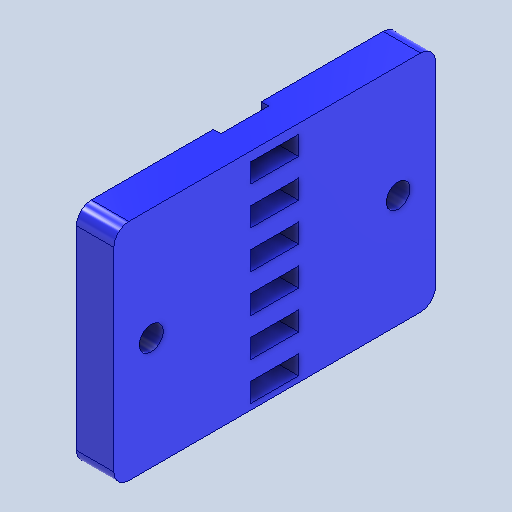
# Autodesk Inventor part: dribl-v3-3DP-3
Saved by Autodesk Inventor 2025.2 (Build 292293000, 293)
## iProperties
Created: 2025-04-20
Part Number: dribl-v3-3DP-3
Material: ABS プラスチック
Document SubType Name: Modeling
Designer: haruy
Density: 1.06 g/cm^3
Appearance: 青 - 壁塗料 - 光沢
Author: haruy
Autodesk Inventor part; units mm, degrees
ref_plane "YZ Plane" through (0, 0, 0) normal (1, 0, 0) x (0, 1, 0)
ref_plane "XZ Plane" through (0, 0, 0) normal (0, 1, 0) x (-1, 0, 0)
ref_plane "XY Plane" through (0, 0, 0) normal (0, 0, 1) x (1, 0, 0)
sketch "スケッチ1" plane through (0, 0, 0) normal (1, 0, 0) x (0, 1, 0)
  line L0 (0, 0) -> (30, 0)
  line L1 (30, 0) -> (30, -43)
  line L2 (30, -43) -> (0, -43)
  line L3 (0, -43) -> (0, 0)
  circle A0 centre (15, -5) radius 1.6
  circle A1 centre (15, -38) radius 1.6
  line L4 (28.75, -18.3) -> (26.18, -18.3)
  line L5 (26.18, -18.3) -> (26.18, -24.7)
  line L6 (26.18, -24.7) -> (28.75, -24.7)
  line L7 (28.75, -24.7) -> (28.75, -18.3)
  line L8 (30, -21.5) -> (0, -21.5)
  line L9 (23.67, -18.3) -> (21.1, -18.3)
  line L10 (21.1, -24.7) -> (23.67, -24.7)
  line L11 (23.67, -24.7) -> (23.67, -18.3)
  line L12 (21.1, -18.3) -> (21.1, -24.7)
  line L13 (18.59, -18.3) -> (16.02, -18.3)
  line L14 (16.02, -24.7) -> (18.59, -24.7)
  line L15 (18.59, -24.7) -> (18.59, -18.3)
  line L16 (16.02, -18.3) -> (16.02, -24.7)
  line L17 (13.51, -18.3) -> (10.94, -18.3)
  line L18 (10.94, -24.7) -> (13.51, -24.7)
  line L19 (13.51, -24.7) -> (13.51, -18.3)
  line L20 (10.94, -18.3) -> (10.94, -24.7)
  line L21 (8.43, -18.3) -> (5.86, -18.3)
  line L22 (5.86, -24.7) -> (8.43, -24.7)
  line L23 (8.43, -24.7) -> (8.43, -18.3)
  line L24 (5.86, -18.3) -> (5.86, -24.7)
  line L25 (3.35, -18.3) -> (0.78, -18.3)
  line L26 (0.78, -24.7) -> (3.35, -24.7)
  line L27 (3.35, -24.7) -> (3.35, -18.3)
  line L28 (0.78, -18.3) -> (0.78, -24.7)
  line L29 (30, -24.7) -> (0, -24.7)
  line L30 (0, -24.7) -> (0, -18.3)
  line L31 (0, -18.3) -> (30, -18.3)
  line L32 (30, -18.3) -> (30, -24.7)
  point P0 (0, -24.7)
  dimension "d0" = 30
  dimension "d1" = 43
  dimension "d2" = 3.2
  dimension "d3" = 3.2
  dimension "d4" = 5
  dimension "d5" = 15
  dimension "d6" = 15
  dimension "d7" = 5
  dimension "d8" = 2.57
  dimension "d9" = 6.4
  dimension "d10" = 3.2
  dimension "d11" = 1.25
  dimension "d14" = 5.08
  dimension "d22" = 0
  dimension "d23" = 0
  constraints: 66 end point, 6 parallel, 4 horizontal, 3 perpendicular, 2 centre point, 2 midpoint, 2 point on line, 40 other
  measures "d0" distance of L1.end L2.end
  measures "d1" distance of L0.end L1.end
  measures "d2" diameter of A0
  measures "d3" diameter of A1
  measures "d4" distance from line of A0.centre L0
  measures "d5" distance from line of A0.centre L3
  measures "d6" distance from line of A1.centre L3
  measures "d7" distance from line of L2 A1.centre
  measures "d8" distance of L6.end L5.end
  measures "d9" distance of L5.end L4.end
  measures "d10" distance between parallel lines of L8 L4
  measures "d11" distance between parallel lines of L7 L1
  measures "d14" distance of L4.start L9.start
  measures "d22" distance between parallel lines of L29 L6
  measures "d23" distance between parallel lines of L4 L31
extrude "押し出し1" add sketch "スケッチ1" along normal blind 5 contours L0 L1 L31 L4 L9 L13 L17 L21 L25 L3 | L31 L28 L8 L3 | L1 L8 L7 L31 | L8 L28 L29 L3 | L1 L29 L7 L8 | L29 L26 L22 L18 L14 L10 L6 L1 L2 L3 | L31 L24 L8 L27 | L5 L8 L11 L31 | L8 L24 L29 L27 | L5 L29 L11 L8 | L31 L20 L8 L23 | L12 L8 L15 L31 | L8 L20 L29 L23 | L12 L29 L15 L8 | L31 L16 L8 L19 | L8 L16 L29 L19
fillet "フィレット1" radius 2 4 edges at (2.5, 30, 0) (2.5, 0, 0) (2.5, 0, -43) (2.5, 30, -43)
extrude "押し出し2" cut sketch "スケッチ1" along normal blind 1 contours L31 L28 L8 L3 | L1 L8 L7 L31 | L8 L28 L29 L3 | L25 L27 L8 L28 | L1 L29 L7 L8 | L7 L8 L5 L4 | L8 L27 L26 L28 | L31 L24 L8 L27 | L7 L6 L5 L8 | L5 L8 L11 L31 | L8 L24 L29 L27 | L21 L23 L8 L24 | L5 L29 L11 L8 | L11 L8 L12 L9 | L8 L23 L22 L24 | L31 L20 L8 L23 | L11 L10 L12 L8 | L12 L8 L15 L31 | L8 L20 L29 L23 | L17 L19 L8 L20 | L12 L29 L15 L8 | L15 L8 L16 L13 | L8 L19 L18 L20 | L31 L16 L8 L19 | L15 L14 L16 L8 | L8 L16 L29 L19
equation "\"d6\" = d5"
equation "\"d7\" = d4"
